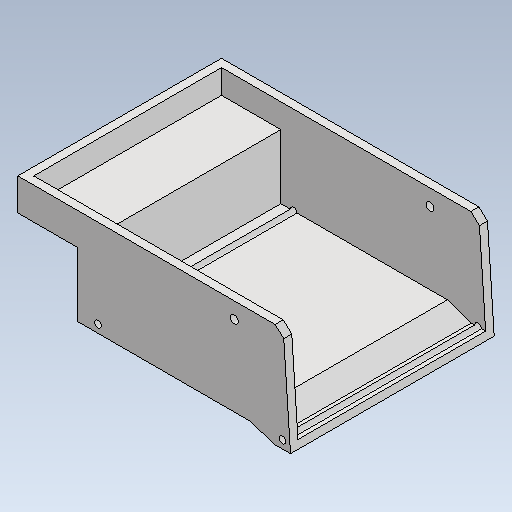
# Autodesk Inventor part: bed
Saved by Autodesk Inventor 2025 (Build 290162000, 162)
## iProperties
Created: 2025-08-20
Part Number: bed
Material: Generic
Document SubType Name: Modeling
Designer: HP
Density: 1 g/cm^3
Appearance: Default
Author: HP
Autodesk Inventor part; units mm, degrees
ref_plane "YZ Plane" through (0, 0, 0) normal (1, 0, 0) x (0, 1, 0)
ref_plane "XZ Plane" through (0, 0, 0) normal (0, 1, 0) x (-1, 0, 0)
sketch "Sketch1" plane through (0, 0, 0) normal (0, 0, 1) x (1, 0, 0)
  line L0 (-85, -15) -> (85, -15)
  line L1 (85, -15) -> (85, 15)
  line L2 (85, 15) -> (-85, 15)
  line L3 (-85, 15) -> (-85, -15)
  line L4 (-85, -15) -> (85, 15) construction
  line L5 (85, -15) -> (-85, 15) construction
  circle A0 centre (-35, -40) radius 2.1
  circle A1 centre (80, -45) radius 2.1
  line L6 (85, -50) -> (75, -50)
  line L7 (75, -50) -> (75, -15) construction
  line L8 (75, -15) -> (85, -15)
  line L9 (85, -15) -> (85, -50)
  line L10 (85, -50) -> (75, -15) construction
  line L11 (75, -50) -> (85, -15) construction
  line L12 (-32.5, -15) -> (-47.5, -15)
  line L13 (-48, -15) -> (75, -15)
  line L14 (75, -45) -> (-48, -45)
  line L15 (-48, -45) -> (-48, -15)
  line L16 (-85, -5) -> (-48, -5)
  line L17 (-48, -5) -> (-48, -15)
  line L18 (85, -50) -> (80.4548, 15)
  line L19 (75, -50) -> (60, -45)
  point P0 (0, 0)
  point P1 (80, -32.5)
  point P2 (85, -15)
  point P3 (12.5, -15)
  point P4 (7.5, -15)
  point P5 (-47.5, -15)
  point P6 (-48, -15)
  point P7 (82.5526, -15)
  dimension "d0" = 170
  dimension "d1" = 30
  dimension "d2" = 4.2
  dimension "d5" = 4.2
  dimension "d7" = 5
  dimension "d10" = 30
  dimension "d14" = 13
  dimension "d15" = 30
  dimension "d18" = 25
  dimension "d19" = 35
  dimension "d20" = 20
  dimension "d21" = 37
  dimension "d36" = 4
  dimension "d43" = 15
  constraints: 38 end point, 5 parallel, 5 point on line, 4 horizontal, 3 midpoint, 3 perpendicular, 2 centre point, 2 collinear, 1 vertical alignment, 4 other
  measures "d0" distance of L2.end L1.end
  measures "d1" distance between parallel lines of L0 L2
  measures "d2" diameter of A0
  measures "d5" diameter of A1
  measures "d7" distance from line of L1 A1.centre
  measures "d10" distance from line of L0 A1.centre
  measures "d14" distance from line of L15 A0.centre
  measures "d15" distance between parallel lines of L13 L14
  measures "d18" distance from line of L0 A0.centre
  measures "d19" distance between parallel lines of L0 L6
  measures "d20" distance between parallel lines of L2 L16
  measures "d21" distance between parallel lines of L15 L3
  measures "d36" angle of L1 L18
  measures "d43" distance from line of L7 L19.end
extrude "Extrusion1" add sketch "Sketch1" along normal blind 127 contours L17 L16 L3 L2 L18 L0 | L0 L18 L6 L19 L14 L15 | A0 | A1
shell "Shell3" thickness 5 removed faces 2 at (83.4849, -28.3333, 42.3333) at (25.3032, 15, 42.3333)
extrude "Extrusion2" cut sketch "Sketch1" along normal blind 25 contours A0 | A1
sketch "Sketch2" plane through (0, 0, 127) normal (0, 0, 1) x (1, 0, 0)
  circle A0 centre (50, 5) radius 2.5
  line L0 (-85, 15) -> (-85, -5) construction
  line L1 (80.4548, 15) -> (-85, 15) construction
  line L2 (-48, -45) -> (60, -45) projected
  line L3 (60, -45) -> (75, -50) projected
  line L4 (75, -50) -> (85, -50) projected
  line L5 (85, -50) -> (80.4548, 15) projected
  line L6 (-85, -5) -> (-48, -5) projected
  line L7 (-48, -5) -> (-48, -45) projected
  point P0 (0, 0)
  dimension "d22" = 5
  dimension "d24" = 10
  constraints: 1 centre point
  measures "d22" diameter of A0
  measures "d24" distance from line of A0.centre L1
ref_plane "Work Plane1" through (0, 0, 63.5) normal (0, 0, -1) x (-1, 0, 0)
mirror "Mirror1" about plane through (0, 0, 63.5) normal (0, 0, -1) of "Extrusion2"
extrude "Extrusion4" cut sketch "Sketch2" against normal through all
chamfer "Chamfer2" distance 5 angle 45 2 edges at (80.4548, 15, 124.5) (80.4548, 15, 2.5)
sketch "Sketch3" plane through (0, 0, 127) normal (0, 0, 1) x (1, 0, 0)
  circle A0 centre (-35, -40) radius 2.1 projected
  circle A1 centre (80, -45) radius 2.1 projected
  point P0 (0, 0)
extrude "Extrusion5" cut sketch "Sketch3" against normal through all
equation "\"d5\" = d2"
body "Solid1"
